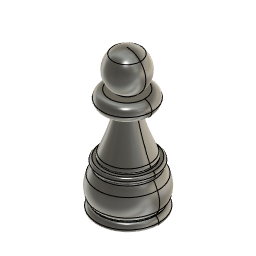
Pawn (Autodesk Fusion 360 design; units mm, degrees)
Autodesk Fusion 360 part; units mm, degrees
sketch "Chess Pieces_SVG" plane through (0, 0, 0) normal (0, 0, 1) x (1, 0, 0)
  spline S0 degree 3 poles (46.9799, 11.3155) (48.9199, 11.5598) (50.8372, 11.3177) (52.7479, 11.3837) knots 0 0 0 0 1 1 1 1
  spline S1 degree 3 poles (52.7479, 11.3837) (53.3742, 11.405) (53.207, 10.9554) (53.1909, 10.673) knots 0 0 0 0 1 1 1 1
  spline S2 degree 3 poles (53.1909, 10.673) (53.1249, 9.5941) (52.9877, 8.5188) (52.9166, 7.4399) knots 0 0 0 0 1 1 1 1
  spline S3 degree 3 poles (52.9166, 7.4399) (52.8748, 6.7959) (52.8682, 6.292) (53.8855, 6.4241) knots 0 0 0 0 1 1 1 1
  spline S4 degree 3 poles (53.8855, 6.4241) (54.6123, 6.5179) (55.4272, 6.4871) (56.1761, 6.4043) knots 0 0 0 0 1 1 1 1
  spline S5 degree 3 poles (56.1761, 6.4043) (57.3592, 6.273) (57.4626, 6.8172) (57.3159, 7.7443) knots 0 0 0 0 1 1 1 1
  spline S6 degree 3 poles (57.3159, 7.7443) (57.1728, 8.6465) (57.1384, 9.567) (56.9858, 10.4669) knots 0 0 0 0 1 1 1 1
  spline S7 degree 3 poles (56.9858, 10.4669) (56.8685, 11.1578) (57.153, 11.4043) (57.7802, 11.4035) knots 0 0 0 0 1 1 1 1
  spline S8 degree 3 poles (57.7802, 11.4035) (59.5097, 11.4013) (61.2406, 11.3984) (62.9687, 11.3881) knots 0 0 0 0 1 1 1 1
  spline S9 degree 3 poles (62.9687, 11.3881) (63.5547, 11.3852) (63.8899, 11.2568) (63.7586, 10.494) knots 0 0 0 0 1 1 1 1
  spline S10 degree 3 poles (63.7586, 10.494) (63.2848, 7.7443) (62.6225, 5.0099) (60.8673, 2.833) knots 0 0 0 0 1 1 1 1
  spline S11 degree 3 poles (60.8673, 2.833) (60.0011, 1.76) (59.1092, 0.4933) (57.0878, 0.5989) knots 0 0 0 0 1 1 1 1
  spline S12 degree 3 poles (57.0878, 0.5989) (52.31, 0.8483) (47.5109, 0.6612) (42.7207, 0.6392) knots 0 0 0 0 1 1 1 1
  spline S13 degree 3 poles (42.7207, 0.6392) (41.996, 0.6363) (41.3528, 0.7749) (40.8247, 1.3177) knots 0 0 0 0 1 1 1 1
  spline S14 degree 3 poles (40.8247, 1.3177) (38.3031, 3.9178) (37.1009, 7.1018) (36.7041, 10.6385) knots 0 0 0 0 1 1 1 1
  spline S15 degree 3 poles (36.7041, 10.6385) (36.6652, 10.9781) (36.5017, 11.4446) (37.1823, 11.4329) knots 0 0 0 0 1 1 1 1
  spline S16 degree 3 poles (37.1823, 11.4329) (38.9551, 11.4021) (40.7293, 11.4072) (42.5029, 11.4028) knots 0 0 0 0 1 1 1 1
  spline S17 degree 3 poles (42.5029, 11.4028) (43.1725, 11.4006) (43.4813, 11.1608) (43.3683, 10.4126) knots 0 0 0 0 1 1 1 1
  spline S18 degree 3 poles (43.3683, 10.4126) (43.2077, 9.3462) (43.1527, 8.2636) (43.0412, 7.1898) knots 0 0 0 0 1 1 1 1
  spline S19 degree 3 poles (43.0412, 7.1898) (42.995, 6.7593) (43.0295, 6.3346) (43.5752, 6.3881) knots 0 0 0 0 1 1 1 1
  spline S20 degree 3 poles (43.5752, 6.3881) (44.7245, 6.5025) (45.8834, 6.2033) (47.0327, 6.5077) knots 0 0 0 0 1 1 1 1
  spline S21 degree 3 poles (47.0327, 6.5077) (47.3239, 6.5854) (47.5476, 6.5473) (47.5058, 6.9477) knots 0 0 0 0 1 1 1 1
  spline S22 degree 3 poles (47.5058, 6.9477) (47.3532, 8.3883) (47.4259, 9.8545) (46.9799, 11.3155) knots 0 0 0 0 1 1 1 1
  spline S23 degree 3 poles (-16.835, 18.1287) (-19.0728, 18.0267) (-21.2409, 20.0423) (-21.3773, 22.3512) knots 0 0 0 0 1 1 1 1
  spline S24 degree 3 poles (-21.3773, 22.3512) (-21.5335, 24.9924) (-19.5642, 27.3219) (-17.0946, 27.415) knots 0 0 0 0 1 1 1 1
  spline S25 degree 3 poles (-17.0946, 27.415) (-14.4762, 27.5133) (-12.0484, 25.742) (-12.0902, 22.4458) knots 0 0 0 0 1 1 1 1
  spline S26 degree 3 poles (-12.0902, 22.4458) (-12.1151, 20.5205) (-13.7082, 18.1778) (-16.835, 18.1287) knots 0 0 0 0 1 1 1 1
  spline S27 degree 3 poles (-58.4766, 30.9107) (-57.8429, 30.1926) (-57.1527, 29.6858) (-56.3202, 29.355) knots 0 0 0 0 1 1 1 1
  spline S28 degree 3 poles (-56.3202, 29.355) (-56.0011, 29.2281) (-55.7122, 29.1797) (-55.443, 29.3382) knots 0 0 0 0 1 1 1 1
  spline S29 degree 3 poles (-55.443, 29.3382) (-55.0704, 29.5597) (-55.1701, 29.9689) (-55.2449, 30.2836) knots 0 0 0 0 1 1 1 1
  spline S30 degree 3 poles (-55.2449, 30.2836) (-55.4078, 30.9679) (-55.7408, 31.5686) (-56.2923, 32.041) knots 0 0 0 0 1 1 1 1
  spline S31 degree 3 poles (-56.2923, 32.041) (-56.7639, 32.4451) (-56.626, 32.7487) (-56.0928, 32.9739) knots 0 0 0 0 1 1 1 1
  spline S32 degree 3 poles (-56.0928, 32.9739) (-55.2889, 33.3128) (-54.4271, 33.4037) (-53.6027, 33.2886) knots 0 0 0 0 1 1 1 1
  spline S33 degree 3 poles (-53.6027, 33.2886) (-52.0837, 33.0751) (-52.0214, 32.8023) (-52.8986, 31.5701) knots 0 0 0 0 1 1 1 1
  spline S34 degree 3 poles (-52.8986, 31.5701) (-53.3313, 30.962) (-54.0589, 30.2198) (-53.3599, 29.5289) knots 0 0 0 0 1 1 1 1
  spline S35 degree 3 poles (-53.3599, 29.5289) (-52.6023, 28.7793) (-51.8387, 29.5912) (-51.2322, 30.0415) knots 0 0 0 0 1 1 1 1
  spline S36 degree 3 poles (-51.2322, 30.0415) (-50.1958, 30.8109) (-49.8841, 30.7889) (-49.6736, 29.5435) knots 0 0 0 0 1 1 1 1
  spline S37 degree 3 poles (-49.6736, 29.5435) (-49.5093, 28.5687) (-49.4088, 27.5617) (-49.876, 26.5899) knots 0 0 0 0 1 1 1 1
  spline S38 degree 3 poles (-49.876, 26.5899) (-50.1459, 26.0288) (-50.3219, 25.7904) (-50.806, 26.405) knots 0 0 0 0 1 1 1 1
  spline S39 degree 3 poles (-50.806, 26.405) (-51.2461, 26.9617) (-51.8607, 27.3219) (-52.5385, 27.5111) knots 0 0 0 0 1 1 1 1
  spline S40 degree 3 poles (-52.5385, 27.5111) (-53.3394, 27.7341) (-53.7281, 27.3373) (-53.5602, 26.5268) knots 0 0 0 0 1 1 1 1
  spline S41 degree 3 poles (-53.5602, 26.5268) (-53.3959, 25.7354) (-52.8597, 25.1611) (-52.3793, 24.5604) knots 0 0 0 0 1 1 1 1
  spline S42 degree 3 poles (-52.3793, 24.5604) (-52.0038, 24.091) (-52.0492, 23.8753) (-52.6837, 23.7118) knots 0 0 0 0 1 1 1 1
  spline S43 degree 3 poles (-52.6837, 23.7118) (-53.7531, 23.4353) (-54.8027, 23.2908) (-55.8706, 23.6604) knots 0 0 0 0 1 1 1 1
  spline S44 degree 3 poles (-55.8706, 23.6604) (-56.5732, 23.9039) (-56.9986, 24.1658) (-56.2278, 24.9102) knots 0 0 0 0 1 1 1 1
  spline S45 degree 3 poles (-56.2278, 24.9102) (-55.8009, 25.3224) (-55.5581, 25.9349) (-55.2713, 26.4777) knots 0 0 0 0 1 1 1 1
  spline S46 degree 3 poles (-55.2713, 26.4777) (-55.1173, 26.7696) (-55.1797, 27.1011) (-55.4004, 27.3453) knots 0 0 0 0 1 1 1 1
  spline S47 degree 3 poles (-55.4004, 27.3453) (-55.6307, 27.6006) (-55.9153, 27.6013) (-56.2432, 27.462) knots 0 0 0 0 1 1 1 1
  spline S48 degree 3 poles (-56.2432, 27.462) (-56.9121, 27.1774) (-57.6118, 26.9617) (-58.101, 26.3698) knots 0 0 0 0 1 1 1 1
  spline S49 degree 3 poles (-58.101, 26.3698) (-58.4898, 25.8997) (-58.7406, 26.0786) (-58.8954, 26.5679) knots 0 0 0 0 1 1 1 1
  spline S50 degree 3 poles (-58.8954, 26.5679) (-59.3538, 28.0194) (-59.4279, 29.4394) (-58.4766, 30.9107) knots 0 0 0 0 1 1 1 1
  spline S51 degree 3 poles (99.919, 0.4038) (97.4773, 2.1487) (95.6341, 4.3579) (94.363, 7.071) knots 0 0 0 0 1 1 1 1
  spline S52 degree 3 poles (94.363, 7.071) (94.0051, 7.8345) (93.6369, 8.6575) (92.9629, 9.1767) knots 0 0 0 0 1 1 1 1
  spline S53 degree 3 poles (92.9629, 9.1767) (92.25, 9.7254) (91.8524, 10.1882) (92.2155, 11.1725) knots 0 0 0 0 1 1 1 1
  spline S54 degree 3 poles (92.2155, 11.1725) (92.5111, 11.9727) (91.9778, 12.7692) (91.3492, 13.1631) knots 0 0 0 0 1 1 1 1
  spline S55 degree 3 poles (91.3492, 13.1631) (90.805, 13.5042) (90.3466, 12.8529) (89.9689, 12.4223) knots 0 0 0 0 1 1 1 1
  spline S56 degree 3 poles (89.9689, 12.4223) (89.5794, 11.98) (89.1525, 11.903) (88.5327, 12.0086) knots 0 0 0 0 1 1 1 1
  spline S57 degree 3 poles (88.5327, 12.0086) (85.3576, 12.5507) (82.3328, 12.0314) (79.4848, 10.5168) knots 0 0 0 0 1 1 1 1
  spline S58 degree 3 poles (79.4848, 10.5168) (76.8142, 9.0968) (75.0488, 6.8935) (73.8092, 4.1731) knots 0 0 0 0 1 1 1 1
  spline S59 degree 3 poles (73.8092, 4.1731) (72.2205, 0.6891) (71.4812, -2.9921) (71.234, -6.7687) knots 0 0 0 0 1 1 1 1
  spline S60 degree 3 poles (71.234, -6.7687) (70.9634, -10.9143) (71.1357, -15.0605) (71.9448, -19.1452) knots 0 0 0 0 1 1 1 1
  spline S61 degree 3 poles (71.9448, -19.1452) (72.379, -21.3368) (72.921, -23.5041) (73.9163, -25.5476) knots 0 0 0 0 1 1 1 1
  spline S62 degree 3 poles (73.9163, -25.5476) (74.2581, -26.2524) (74.6674, -26.606) (75.2769, -26.7262) knots 0 0 0 0 1 1 1 1
  line L0 (75.2769, -26.7262) -> (92.9848, -26.7262)
  spline S63 degree 3 poles (92.9848, -26.7262) (93.4601, -26.6272) (93.6552, -26.314) (93.7176, -25.7331) knots 0 0 0 0 1 1 1 1
  spline S64 degree 3 poles (93.7176, -25.7331) (93.9603, -23.5225) (94.2229, -21.3148) (94.5097, -19.1107) knots 0 0 0 0 1 1 1 1
  spline S65 degree 3 poles (94.5097, -19.1107) (94.5933, -18.4711) (94.4034, -18.0428) (93.9273, -17.5968) knots 0 0 0 0 1 1 1 1
  spline S66 degree 3 poles (93.9273, -17.5968) (91.7548, -15.5695) (89.7429, -13.4014) (88.32, -10.7522) knots 0 0 0 0 1 1 1 1
  spline S67 degree 3 poles (88.32, -10.7522) (86.889, -8.0846) (85.7712, -5.3238) (85.6707, -2.244) knots 0 0 0 0 1 1 1 1
  spline S68 degree 3 poles (85.6707, -2.244) (85.6546, -1.7716) (85.7595, -1.1423) (86.1636, -1.1064) knots 0 0 0 0 1 1 1 1
  spline S69 degree 3 poles (86.1636, -1.1064) (86.7049, -1.058) (86.5788, -1.7254) (86.6536, -2.1149) knots 0 0 0 0 1 1 1 1
  spline S70 degree 3 poles (86.6536, -2.1149) (87.1362, -4.6461) (88.5569, -5.4544) (91.102, -4.8412) knots 0 0 0 0 1 1 1 1
  spline S71 degree 3 poles (91.102, -4.8412) (93.3112, -4.3094) (95.5358, -3.9522) (97.3974, -5.9245) knots 0 0 0 0 1 1 1 1
  spline S72 degree 3 poles (97.3974, -5.9245) (97.6423, -6.1842) (98.4506, -6.8971) (99.1004, -5.8336) knots 0 0 0 0 1 1 1 1
  spline S73 degree 3 poles (99.1004, -5.8336) (99.6373, -4.9578) (100.3305, -4.1679) (100.7713, -3.2144) knots 0 0 0 0 1 1 1 1
  spline S74 degree 3 poles (100.7713, -3.2144) (101.5238, -1.5875) (101.3529, -0.6216) (99.919, 0.4038) knots 0 0 0 0 1 1 1 1
  line L1 (63.1256, -42.2624) -> (37.0606, -42.2624)
  spline S75 degree 3 poles (37.0606, -42.2624) (36.253, -42.5485) (35.832, -43.2511) (35.4088, -44.5662) knots 0 0 0 0 1 1 1 1
  spline S76 degree 3 poles (35.4088, -44.5662) (35.1081, -45.5014) (35.3692, -45.6166) (36.1687, -45.6144) knots 0 0 0 0 1 1 1 1
  spline S77 degree 3 poles (36.1687, -45.6144) (40.4983, -45.5982) (44.8279, -45.599) (49.1568, -45.6019) knots 0 0 0 0 1 1 1 1
  spline S78 degree 3 poles (49.1568, -45.6019) (54.1972, -45.6056) (59.2353, -45.6041) (64.2735, -45.6378) knots 0 0 0 0 1 1 1 1
  spline S79 degree 3 poles (64.2735, -45.6378) (65.0876, -45.6437) (65.169, -45.3056) (65.0179, -44.6381) knots 0 0 0 0 1 1 1 1
  spline S80 degree 3 poles (65.0179, -44.6381) (64.7048, -43.2585) (64.1495, -42.5323) (63.1256, -42.2624) knots 0 0 0 0 1 1 1 1
  spline S81 degree 3 poles (-9.7204, -27.3922) (-9.6412, -27.39) (-9.562, -27.3864) (-9.4828, -27.3819) knots 0 0 0 0 1 1 1 1
  spline S82 degree 3 poles (-9.4828, -27.3819) (-9.4828, -27.3856) (-9.4828, -27.3893) (-9.4828, -27.3922) knots 0 0 0 0 1 1 1 1
  line L2 (-9.4828, -27.3922) -> (-6.4902, -27.3922)
  spline S83 degree 3 poles (-6.4902, -27.3922) (-6.0927, -26.4563) (-6.9325, -25.981) (-7.2743, -25.3554) knots 0 0 0 0 1 1 1 1
  spline S84 degree 3 poles (-7.2743, -25.3554) (-9.9023, -20.5556) (-11.3949, -15.4251) (-12.0169, -9.9989) knots 0 0 0 0 1 1 1 1
  spline S85 degree 3 poles (-12.0169, -9.9989) (-12.1592, -8.7557) (-12.0425, -7.4707) (-12.4922, -6.1409) knots 0 0 0 0 1 1 1 1
  line L3 (-12.4922, -6.1409) -> (-21.2754, -6.1409)
  spline S86 degree 3 poles (-21.2754, -6.1409) (-21.4712, -6.3697) (-21.5394, -6.6815) (-21.56, -7.0724) knots 0 0 0 0 1 1 1 1
  spline S87 degree 3 poles (-21.56, -7.0724) (-21.7338, -10.3744) (-22.2787, -13.6259) (-23.0415, -16.8392) knots 0 0 0 0 1 1 1 1
  spline S88 degree 3 poles (-23.0415, -16.8392) (-23.9342, -20.6055) (-26.0055, -23.8782) (-27.4981, -27.3922) knots 0 0 0 0 1 1 1 1
  line L4 (-27.4981, -27.3922) -> (-9.7204, -27.3922)
  spline S89 degree 3 poles (-5.968, -27.8162) (-6.0443, -27.811) (-6.155, -27.8132) (-6.2621, -27.8088) knots 0 0 0 0 1 1 1 1
  line L5 (-6.2621, -27.8088) -> (-27.8971, -27.8088)
  spline S90 degree 3 poles (-27.8971, -27.8088) (-27.9741, -27.8257) (-28.0562, -27.8316) (-28.1376, -27.8323) knots 0 0 0 0 1 1 1 1
  spline S91 degree 3 poles (-28.1376, -27.8323) (-29.0031, -27.8404) (-29.3339, -28.4902) (-29.2965, -29.1269) knots 0 0 0 0 1 1 1 1
  spline S92 degree 3 poles (-29.2965, -29.1269) (-29.2488, -29.9183) (-28.6371, -30.1772) (-27.7995, -30.1742) knots 0 0 0 0 1 1 1 1
  spline S93 degree 3 poles (-27.7995, -30.1742) (-20.5837, -30.15) (-13.3672, -30.1698) (-6.1514, -30.1882) knots 0 0 0 0 1 1 1 1
  spline S94 degree 3 poles (-6.1514, -30.1882) (-5.426, -30.1896) (-4.76, -30.0261) (-4.6661, -29.2383) knots 0 0 0 0 1 1 1 1
  spline S95 degree 3 poles (-4.6661, -29.2383) (-4.5642, -28.3765) (-5.0614, -27.8697) (-5.968, -27.8162) knots 0 0 0 0 1 1 1 1
  line L6 (41.1782, -2.9745) -> (58.8041, -2.9745)
  spline S96 degree 3 poles (58.8041, -2.9745) (58.8781, -2.9665) (58.9508, -2.9599) (59.0241, -2.9481) knots 0 0 0 0 1 1 1 1
  spline S97 degree 3 poles (59.0241, -2.9481) (59.9871, -2.7992) (60.7734, -1.9176) (60.6392, -1.1401) knots 0 0 0 0 1 1 1 1
  spline S98 degree 3 poles (60.6392, -1.1401) (60.4712, -0.1646) (59.8867, 0.2996) (58.8664, 0.2952) knots 0 0 0 0 1 1 1 1
  spline S99 degree 3 poles (58.8664, 0.2952) (53.1557, 0.2659) (47.4449, 0.2534) (41.7349, 0.2534) knots 0 0 0 0 1 1 1 1
  spline S100 degree 3 poles (41.7349, 0.2534) (40.9839, 0.2534) (40.3597, 0.0701) (40.0465, -0.6458) knots 0 0 0 0 1 1 1 1
  spline S101 degree 3 poles (40.0465, -0.6458) (39.616, -1.6301) (40.1822, -2.6393) (41.1782, -2.9745) knots 0 0 0 0 1 1 1 1
  spline S102 degree 3 poles (59.6659, -16.058) (59.2441, -12.3526) (58.9089, -8.642) (58.5584, -4.9314) knots 0 0 0 0 1 1 1 1
  spline S103 degree 3 poles (58.5584, -4.9314) (58.4579, -3.865) (58.4051, -3.507) (57.8894, -3.3911) knots 0 0 0 0 1 1 1 1
  line L7 (57.8894, -3.3911) -> (42.4677, -3.3911)
  spline S104 degree 3 poles (42.4677, -3.3911) (42.2373, -3.4711) (42.0672, -3.6647) (42.0312, -4.1385) knots 0 0 0 0 1 1 1 1
  spline S105 degree 3 poles (42.0312, -4.1385) (41.8523, -6.6015) (41.5948, -9.0593) (41.3565, -11.5172) knots 0 0 0 0 1 1 1 1
  spline S106 degree 3 poles (41.3565, -11.5172) (40.9729, -15.4676) (40.5775, -19.4165) (40.18, -23.4565) knots 0 0 0 0 1 1 1 1
  spline S107 degree 3 poles (40.18, -23.4565) (42.2982, -23.4565) (44.4539, -23.4535) (46.611, -23.4565) knots 0 0 0 0 1 1 1 1
  spline S108 degree 3 poles (46.611, -23.4565) (50.7448, -23.4609) (54.8778, -23.4425) (59.0102, -23.4924) knots 0 0 0 0 1 1 1 1
  spline S109 degree 3 poles (59.0102, -23.4924) (59.993, -23.5049) (60.268, -23.1792) (60.1947, -22.2242) knots 0 0 0 0 1 1 1 1
  spline S110 degree 3 poles (60.1947, -22.2242) (60.0385, -20.1661) (59.8984, -18.0934) (59.6659, -16.058) knots 0 0 0 0 1 1 1 1
  line L8 (-64.3963, -26.9763) -> (-44.2056, -26.9763)
  spline S111 degree 3 poles (-44.2056, -26.9763) (-44.1359, -26.2238) (-44.6031, -25.6231) (-44.9134, -25.0349) knots 0 0 0 0 1 1 1 1
  spline S112 degree 3 poles (-44.9134, -25.0349) (-47.8142, -19.5361) (-49.5335, -13.7102) (-49.9669, -7.5059) knots 0 0 0 0 1 1 1 1
  spline S113 degree 3 poles (-49.9669, -7.5059) (-50.0792, -5.8959) (-50.1114, -5.5856) (-51.1735, -5.4492) knots 0 0 0 0 1 1 1 1
  line L9 (-51.1735, -5.4492) -> (-58.6922, -5.4492)
  spline S114 degree 3 poles (-58.6922, -5.4492) (-58.9497, -5.5204) (-59.1543, -5.6891) (-59.1565, -6.0976) knots 0 0 0 0 1 1 1 1
  spline S115 degree 3 poles (-59.1565, -6.0976) (-59.1587, -6.7159) (-59.3619, -7.3247) (-59.3736, -7.9151) knots 0 0 0 0 1 1 1 1
  spline S116 degree 3 poles (-59.3736, -7.9151) (-59.4381, -11.1314) (-60.1151, -14.239) (-60.8882, -17.3342) knots 0 0 0 0 1 1 1 1
  spline S117 degree 3 poles (-60.8882, -17.3342) (-61.6239, -20.2784) (-63.0849, -22.9386) (-64.2071, -25.7309) knots 0 0 0 0 1 1 1 1
  spline S118 degree 3 poles (-64.2071, -25.7309) (-64.3941, -26.1959) (-64.7191, -26.6646) (-64.3963, -26.9763) knots 0 0 0 0 1 1 1 1
  line L10 (-65.374, -29.7708) -> (-43.1949, -29.7708)
  spline S119 degree 3 poles (-43.1949, -29.7708) (-42.7805, -29.5999) (-42.5098, -29.22) (-42.4313, -28.7433) knots 0 0 0 0 1 1 1 1
  spline S120 degree 3 poles (-42.4313, -28.7433) (-42.3272, -28.1037) (-42.9543, -27.6211) (-43.6592, -27.4274) knots 0 0 0 0 1 1 1 1
  spline S121 degree 3 poles (-43.6592, -27.4274) (-43.7472, -27.4025) (-43.8755, -27.4135) (-43.987, -27.3929) knots 0 0 0 0 1 1 1 1
  line L11 (-43.987, -27.3929) -> (-64.9017, -27.3929)
  spline S122 degree 3 poles (-64.9017, -27.3929) (-64.9208, -27.3952) (-64.9406, -27.3959) (-64.9604, -27.3973) knots 0 0 0 0 1 1 1 1
  spline S123 degree 3 poles (-64.9604, -27.3973) (-65.7951, -27.4487) (-66.2799, -27.935) (-66.2564, -28.7271) knots 0 0 0 0 1 1 1 1
  spline S124 degree 3 poles (-66.2564, -28.7271) (-66.2373, -29.3352) (-65.8985, -29.6608) (-65.374, -29.7708) knots 0 0 0 0 1 1 1 1
  line L12 (-66.5674, -42.3248) -> (-42.8223, -42.3248)
  spline S125 degree 3 poles (-42.8223, -42.3248) (-42.314, -42.2052) (-41.9465, -41.9074) (-41.6509, -41.3067) knots 0 0 0 0 1 1 1 1
  spline S126 degree 3 poles (-41.6509, -41.3067) (-40.1246, -38.2101) (-40.5889, -35.2337) (-42.1504, -32.3475) knots 0 0 0 0 1 1 1 1
  spline S127 degree 3 poles (-42.1504, -32.3475) (-42.5553, -31.5994) (-42.7607, -30.5762) (-43.5858, -30.1874) knots 0 0 0 0 1 1 1 1
  line L13 (-43.5858, -30.1874) -> (-59.2379, -30.1874)
  spline S128 degree 3 poles (-59.2379, -30.1874) (-60.0528, -30.2124) (-60.8669, -30.227) (-61.6752, -30.1874) knots 0 0 0 0 1 1 1 1
  line L14 (-61.6752, -30.1874) -> (-64.4932, -30.1874)
  spline S129 degree 3 poles (-64.4932, -30.1874) (-65.6454, -30.4683) (-66.4698, -31.2502) (-67.1857, -32.5983) knots 0 0 0 0 1 1 1 1
  spline S130 degree 3 poles (-67.1857, -32.5983) (-68.7898, -35.6195) (-68.9159, -38.5086) (-67.4057, -41.5378) knots 0 0 0 0 1 1 1 1
  spline S131 degree 3 poles (-67.4057, -41.5378) (-67.1908, -41.9712) (-66.9246, -42.2148) (-66.5674, -42.3248) knots 0 0 0 0 1 1 1 1
  line L15 (-42.512, -42.7392) -> (-66.5989, -42.7392)
  spline S132 degree 3 poles (-66.5989, -42.7392) (-67.6221, -42.9335) (-68.3072, -43.8474) (-68.1319, -45.0239) knots 0 0 0 0 1 1 1 1
  spline S133 degree 3 poles (-68.1319, -45.0239) (-67.9602, -46.1857) (-66.9378, -45.4545) (-66.307, -45.6063) knots 0 0 0 0 1 1 1 1
  spline S134 degree 3 poles (-66.307, -45.6063) (-66.1258, -45.6518) (-65.9241, -45.6158) (-65.7312, -45.6158) knots 0 0 0 0 1 1 1 1
  spline S135 degree 3 poles (-65.7312, -45.6158) (-58.0277, -45.618) (-50.3227, -45.6283) (-42.6184, -45.5931) knots 0 0 0 0 1 1 1 1
  spline S136 degree 3 poles (-42.6184, -45.5931) (-42.1387, -45.5909) (-41.4309, -45.9364) (-41.1515, -45.321) knots 0 0 0 0 1 1 1 1
  spline S137 degree 3 poles (-41.1515, -45.321) (-40.8654, -44.6924) (-41.2021, -44.0521) (-41.5343, -43.4638) knots 0 0 0 0 1 1 1 1
  spline S138 degree 3 poles (-41.5343, -43.4638) (-41.7837, -43.023) (-42.1196, -42.825) (-42.512, -42.7392) knots 0 0 0 0 1 1 1 1
  line L16 (6.5148, -28.0846) -> (26.022, -28.0846)
  spline S139 degree 3 poles (26.022, -28.0846) (26.7576, -27.8235) (27.0576, -27.214) (26.8706, -26.5348) knots 0 0 0 0 1 1 1 1
  spline S140 degree 3 poles (26.8706, -26.5348) (26.6799, -25.8431) (26.0865, -25.4661) (25.2636, -25.4735) knots 0 0 0 0 1 1 1 1
  spline S141 degree 3 poles (25.2636, -25.4735) (21.7877, -25.5013) (18.3111, -25.4852) (14.8345, -25.483) knots 0 0 0 0 1 1 1 1
  spline S142 degree 3 poles (14.8345, -25.483) (12.285, -25.4823) (9.7354, -25.4691) (7.1859, -25.4749) knots 0 0 0 0 1 1 1 1
  spline S143 degree 3 poles (7.1859, -25.4749) (6.2346, -25.4779) (5.7425, -26.0412) (5.741, -26.9345) knots 0 0 0 0 1 1 1 1
  spline S144 degree 3 poles (5.741, -26.9345) (5.7388, -27.5763) (6.0358, -27.935) (6.5148, -28.0846) knots 0 0 0 0 1 1 1 1
  line L17 (38.6661, -26.6969) -> (40.1506, -26.6969)
  spline S145 degree 3 poles (40.1506, -26.6969) (40.1675, -26.6969) (40.1837, -26.6969) (40.2005, -26.6969) knots 0 0 0 0 1 1 1 1
  line L18 (40.2005, -26.6969) -> (61.3807, -26.6969)
  spline S146 degree 3 poles (61.3807, -26.6969) (62.4384, -26.5781) (63.0156, -26.0867) (62.9833, -25.3275) knots 0 0 0 0 1 1 1 1
  spline S147 degree 3 poles (62.9833, -25.3275) (62.9437, -24.3931) (62.2066, -23.8819) (60.8878, -23.8775) knots 0 0 0 0 1 1 1 1
  spline S148 degree 3 poles (60.8878, -23.8775) (59.1591, -23.8701) (57.4288, -23.8687) (55.7, -23.8643) knots 0 0 0 0 1 1 1 1
  spline S149 degree 3 poles (55.7, -23.8643) (51.5134, -23.8569) (47.3276, -23.8452) (43.1402, -23.8437) knots 0 0 0 0 1 1 1 1
  spline S150 degree 3 poles (43.1402, -23.8437) (41.8765, -23.8415) (40.6142, -23.8643) (39.3504, -23.8789) knots 0 0 0 0 1 1 1 1
  spline S151 degree 3 poles (39.3504, -23.8789) (38.3324, -23.8914) (37.83, -24.5508) (37.8234, -25.4273) knots 0 0 0 0 1 1 1 1
  spline S152 degree 3 poles (37.8234, -25.4273) (37.8182, -26.0705) (38.1013, -26.5297) (38.6661, -26.6969) knots 0 0 0 0 1 1 1 1
  spline S153 degree 3 poles (64.8793, -32.5367) (64.173, -30.8028) (63.0933, -29.2941) (62.2125, -27.6673) knots 0 0 0 0 1 1 1 1
  spline S154 degree 3 poles (62.2125, -27.6673) (61.944, -27.1715) (61.4944, -27.137) (61.0176, -27.1377) knots 0 0 0 0 1 1 1 1
  spline S155 degree 3 poles (61.0176, -27.1377) (59.6673, -27.1377) (58.3163, -27.1384) (56.966, -27.1384) knots 0 0 0 0 1 1 1 1
  spline S156 degree 3 poles (56.966, -27.1384) (55.6795, -27.1392) (54.3937, -27.1384) (53.108, -27.1384) knots 0 0 0 0 1 1 1 1
  spline S157 degree 3 poles (53.108, -27.1384) (53.108, -27.1297) (53.108, -27.1223) (53.108, -27.1135) knots 0 0 0 0 1 1 1 1
  line L19 (53.108, -27.1135) -> (39.5052, -27.1135)
  spline S158 degree 3 poles (39.5052, -27.1135) (39.335, -27.1487) (39.1832, -27.2279) (39.0629, -27.404) knots 0 0 0 0 1 1 1 1
  spline S159 degree 3 poles (39.0629, -27.404) (37.8916, -29.1173) (36.6594, -30.8065) (35.6729, -32.6255) knots 0 0 0 0 1 1 1 1
  spline S160 degree 3 poles (35.6729, -32.6255) (34.4663, -34.8515) (34.9013, -37.2177) (35.7132, -39.4635) knots 0 0 0 0 1 1 1 1
  spline S161 degree 3 poles (35.7132, -39.4635) (36.2743, -41.0163) (36.63, -41.5752) (37.6041, -41.7417) knots 0 0 0 0 1 1 1 1
  line L20 (37.6041, -41.7417) -> (63.1872, -41.7417)
  spline S162 degree 3 poles (63.1872, -41.7417) (63.4351, -41.6471) (63.6603, -41.4688) (63.8408, -41.1446) knots 0 0 0 0 1 1 1 1
  spline S163 degree 3 poles (63.8408, -41.1446) (65.3576, -38.4198) (66.1372, -35.6239) (64.8793, -32.5367) knots 0 0 0 0 1 1 1 1
  spline S164 degree 3 poles (-4.7835, -42.4612) (-3.6312, -42.0248) (-3.409, -40.7698) (-3.1075, -39.6946) knots 0 0 0 0 1 1 1 1
  spline S165 degree 3 poles (-3.1075, -39.6946) (-2.2376, -36.5891) (-3.4258, -33.8804) (-4.9507, -31.2598) knots 0 0 0 0 1 1 1 1
  spline S166 degree 3 poles (-4.9507, -31.2598) (-5.3277, -30.6107) (-5.7641, -30.4222) (-6.5276, -30.4265) knots 0 0 0 0 1 1 1 1
  spline S167 degree 3 poles (-6.5276, -30.4265) (-13.563, -30.4662) (-20.5984, -30.4625) (-27.6337, -30.417) knots 0 0 0 0 1 1 1 1
  spline S168 degree 3 poles (-27.6337, -30.417) (-28.3305, -30.4126) (-28.7831, -30.6547) (-29.0662, -31.1615) knots 0 0 0 0 1 1 1 1
  spline S169 degree 3 poles (-29.0662, -31.1615) (-29.6508, -32.2103) (-30.4414, -33.122) (-30.894, -34.267) knots 0 0 0 0 1 1 1 1
  spline S170 degree 3 poles (-30.894, -34.267) (-32.0653, -37.2279) (-31.546, -39.9058) (-29.8752, -42.4612) knots 0 0 0 0 1 1 1 1
  line L21 (-29.8752, -42.4612) -> (-4.7835, -42.4612)
  line L22 (-4.493, -42.8785) -> (-29.9911, -42.8785)
  spline S171 degree 3 poles (-29.9911, -42.8785) (-30.1803, -43.0326) (-30.3784, -43.1939) (-30.5683, -43.3685) knots 0 0 0 0 1 1 1 1
  spline S172 degree 3 poles (-30.5683, -43.3685) (-31.1434, -43.8937) (-31.2974, -44.6513) (-31.0942, -45.2843) knots 0 0 0 0 1 1 1 1
  spline S173 degree 3 poles (-31.0942, -45.2843) (-30.8999, -45.8938) (-30.1473, -45.5821) (-29.65, -45.5872) knots 0 0 0 0 1 1 1 1
  spline S174 degree 3 poles (-29.65, -45.5872) (-26.3355, -45.6195) (-23.021, -45.6224) (-19.7058, -45.618) knots 0 0 0 0 1 1 1 1
  spline S175 degree 3 poles (-19.7058, -45.618) (-14.4857, -45.6107) (-9.2664, -45.5711) (-4.0471, -45.5997) knots 0 0 0 0 1 1 1 1
  spline S176 degree 3 poles (-4.0471, -45.5997) (-3.0914, -45.6056) (-3.1141, -45.2777) (-3.2329, -44.4995) knots 0 0 0 0 1 1 1 1
  spline S177 degree 3 poles (-3.2329, -44.4995) (-3.3759, -43.5563) (-3.8483, -43.1147) (-4.493, -42.8785) knots 0 0 0 0 1 1 1 1
  line L23 (74.0652, -29.5464) -> (94.1723, -29.5464)
  spline S178 degree 3 poles (94.1723, -29.5464) (94.6586, -29.2405) (95.0518, -28.8305) (94.7936, -28.0861) knots 0 0 0 0 1 1 1 1
  spline S179 degree 3 poles (94.7936, -28.0861) (94.4753, -27.17) (93.6853, -27.1216) (92.888, -27.123) knots 0 0 0 0 1 1 1 1
  spline S180 degree 3 poles (92.888, -27.123) (92.7325, -27.123) (92.5793, -27.1289) (92.4238, -27.1274) knots 0 0 0 0 1 1 1 1
  spline S181 degree 3 poles (92.4238, -27.1274) (88.5716, -27.123) (84.718, -27.1113) (80.8651, -27.1135) knots 0 0 0 0 1 1 1 1
  spline S182 degree 3 poles (80.8651, -27.1135) (78.8576, -27.1142) (76.8502, -27.1436) (74.8427, -27.1487) knots 0 0 0 0 1 1 1 1
  spline S183 degree 3 poles (74.8427, -27.1487) (73.9354, -27.1494) (73.2753, -27.5536) (73.2701, -28.4711) knots 0 0 0 0 1 1 1 1
  spline S184 degree 3 poles (73.2701, -28.4711) (73.2672, -29.0873) (73.6009, -29.4012) (74.0652, -29.5464) knots 0 0 0 0 1 1 1 1
  spline S185 degree 3 poles (94.2758, -42.6996) (93.0516, -42.7003) (91.8275, -42.6996) (90.6033, -42.6996) knots 0 0 0 0 1 1 1 1
  spline S186 degree 3 poles (90.6033, -42.6996) (90.6033, -42.6966) (90.6033, -42.6952) (90.6033, -42.6922) knots 0 0 0 0 1 1 1 1
  line L24 (90.6033, -42.6922) -> (76.6477, -42.6922)
  spline S187 degree 3 poles (76.6477, -42.6922) (76.1483, -42.7275) (75.6495, -42.7568) (75.1559, -42.6922) knots 0 0 0 0 1 1 1 1
  line L25 (75.1559, -42.6922) -> (73.5437, -42.6922)
  spline S188 degree 3 poles (73.5437, -42.6922) (73.4814, -42.704) (73.4117, -42.704) (73.3362, -42.6922) knots 0 0 0 0 1 1 1 1
  line L26 (73.3347, -42.6922) -> (72.8704, -42.6922)
  spline S189 degree 3 poles (72.8704, -42.6922) (72.2536, -42.7964) (71.9316, -43.3318) (71.6741, -43.865) knots 0 0 0 0 1 1 1 1
  spline S190 degree 3 poles (71.6741, -43.865) (71.0881, -45.0723) (71.4849, -45.6232) (72.8125, -45.5953) knots 0 0 0 0 1 1 1 1
  spline S191 degree 3 poles (72.8125, -45.5953) (73.4286, -45.5813) (74.0454, -45.596) (74.6623, -45.596) knots 0 0 0 0 1 1 1 1
  spline S192 degree 3 poles (74.6623, -45.596) (81.5282, -45.5997) (88.3956, -45.6026) (95.2623, -45.5997) knots 0 0 0 0 1 1 1 1
  spline S193 degree 3 poles (95.2623, -45.5997) (95.6246, -45.599) (96.0456, -45.7127) (96.1791, -45.1552) knots 0 0 0 0 1 1 1 1
  spline S194 degree 3 poles (96.1791, -45.1552) (96.4527, -44.0191) (95.4427, -42.6974) (94.2758, -42.6996) knots 0 0 0 0 1 1 1 1
  line L27 (93.9941, -29.963) -> (74.286, -29.963)
  spline S195 degree 3 poles (74.286, -29.963) (73.8004, -30.1904) (73.4425, -30.6664) (73.0912, -31.2312) knots 0 0 0 0 1 1 1 1
  spline S196 degree 3 poles (73.0912, -31.2312) (72.7098, -31.8443) (72.4157, -32.4854) (72.0929, -33.1184) knots 0 0 0 0 1 1 1 1
  spline S197 degree 3 poles (72.0929, -33.1184) (70.714, -35.805) (70.8593, -38.488) (72.0665, -41.1975) knots 0 0 0 0 1 1 1 1
  spline S198 degree 3 poles (72.0665, -41.1975) (72.3057, -41.7365) (72.5902, -42.126) (73.0112, -42.2756) knots 0 0 0 0 1 1 1 1
  line L28 (73.0112, -42.2756) -> (73.9053, -42.2756)
  spline S199 degree 3 poles (73.9053, -42.2756) (73.909, -42.2756) (73.9127, -42.2742) (73.9141, -42.2734) knots 0 0 0 0 1 1 1 1
  spline S200 degree 3 poles (73.9141, -42.2734) (73.9149, -42.2727) (73.9149, -42.2705) (73.9149, -42.269) knots 0 0 0 0 1 1 1 1
  spline S201 degree 3 poles (73.9149, -42.269) (73.9185, -42.2705) (73.9207, -42.2727) (73.9229, -42.2734) knots 0 0 0 0 1 1 1 1
  spline S202 degree 3 poles (73.9229, -42.2734) (75.3781, -42.2734) (76.8333, -42.2734) (78.2885, -42.2734) knots 0 0 0 0 1 1 1 1
  spline S203 degree 2 poles (78.2885, -42.2734) (78.2885, -42.2742) (78.2885, -42.2756) knots 0 0 0 1 1 1
  line L29 (78.2885, -42.2756) -> (94.6872, -42.2756)
  spline S204 degree 3 poles (94.6872, -42.2756) (95.0246, -42.1744) (95.2696, -41.9478) (95.4508, -41.5833) knots 0 0 0 0 1 1 1 1
  spline S205 degree 3 poles (95.4508, -41.5833) (95.9869, -40.5109) (96.4322, -39.4247) (96.5253, -38.1866) knots 0 0 0 0 1 1 1 1
  spline S206 degree 3 poles (96.5253, -38.1866) (96.7541, -35.1134) (95.6114, -32.5081) (93.9941, -29.963) knots 0 0 0 0 1 1 1 1
  line L30 (73.9134, -42.2734) -> (73.9134, -42.2756)
  line L31 (73.9134, -42.2756) -> (73.9259, -42.2756)
  line L32 (73.9259, -42.2756) -> (73.9215, -42.2734)
  line L33 (73.9215, -42.2734) -> (73.9141, -42.2734)
  line L34 (73.9141, -42.2734) -> (73.9134, -42.2734)
  spline S207 degree 3 poles (21.9417, 0.0275) (21.3835, 0.5285) (21.6058, 0.7185) (21.9043, 1.1981) knots 0 0 0 0 1 1 1 1
  spline S208 degree 3 poles (21.9043, 1.1981) (23.4922, 3.7469) (24.0856, 6.3698) (22.5145, 9.212) knots 0 0 0 0 1 1 1 1
  spline S209 degree 3 poles (22.5145, 9.212) (21.1547, 11.672) (19.6247, 14.011) (17.9451, 16.2569) knots 0 0 0 0 1 1 1 1
  spline S210 degree 3 poles (17.9451, 16.2569) (17.6972, 16.5869) (17.5629, 16.8502) (17.6451, 17.1583) knots 0 0 0 0 1 1 1 1
  spline S211 degree 3 poles (17.6451, 17.1583) (18.2913, 17.5808) (18.7196, 18.3098) (18.7196, 19.1401) knots 0 0 0 0 1 1 1 1
  spline S212 degree 3 poles (18.7196, 19.1401) (18.7196, 20.4479) (17.6605, 21.5077) (16.352, 21.5077) knots 0 0 0 0 1 1 1 1
  spline S213 degree 3 poles (16.352, 21.5077) (15.0435, 21.5077) (13.9844, 20.4479) (13.9844, 19.1401) knots 0 0 0 0 1 1 1 1
  spline S214 degree 3 poles (13.9844, 19.1401) (13.9844, 18.315) (14.4076, 17.5888) (15.0472, 17.1656) knots 0 0 0 0 1 1 1 1
  spline S215 degree 3 poles (15.0472, 17.1656) (15.1059, 16.6287) (14.7303, 16.196) (14.3753, 15.7046) knots 0 0 0 0 1 1 1 1
  spline S216 degree 3 poles (14.3753, 15.7046) (14.1039, 15.329) (13.848, 14.9396) (13.548, 14.5875) knots 0 0 0 0 1 1 1 1
  spline S217 degree 3 poles (13.548, 14.5875) (12.9253, 13.8592) (12.8197, 13.1433) (13.3089, 12.261) knots 0 0 0 0 1 1 1 1
  spline S218 degree 3 poles (13.3089, 12.261) (13.848, 11.2847) (14.2543, 10.2322) (14.6988, 9.2046) knots 0 0 0 0 1 1 1 1
  spline S219 degree 3 poles (14.6988, 9.2046) (14.7963, 8.9794) (14.9892, 8.6567) (14.6196, 8.5086) knots 0 0 0 0 1 1 1 1
  spline S220 degree 3 poles (14.6196, 8.5086) (14.3108, 8.3853) (14.1259, 8.6479) (13.9947, 8.8914) knots 0 0 0 0 1 1 1 1
  spline S221 degree 3 poles (13.9947, 8.8914) (13.8868, 9.0953) (13.8318, 9.3308) (13.7115, 9.5273) knots 0 0 0 0 1 1 1 1
  spline S222 degree 3 poles (13.7115, 9.5273) (13.1592, 10.4244) (12.9935, 11.537) (12.2204, 12.3614) knots 0 0 0 0 1 1 1 1
  spline S223 degree 3 poles (12.2204, 12.3614) (11.8119, 11.8333) (11.3953, 11.4175) (11.1268, 10.9217) knots 0 0 0 0 1 1 1 1
  spline S224 degree 3 poles (11.1268, 10.9217) (10.2679, 9.3322) (9.0467, 7.924) (9.2, 5.8798) knots 0 0 0 0 1 1 1 1
  spline S225 degree 3 poles (9.2, 5.8798) (9.3394, 4.0418) (9.965, 2.4582) (10.964, 0.9744) knots 0 0 0 0 1 1 1 1
  spline S226 degree 3 poles (10.964, 0.9744) (11.1224, 0.7397) (11.2977, 0.6011) (11.0857, 0.285) knots 0 0 0 0 1 1 1 1
  spline S227 degree 3 poles (11.0857, 0.285) (10.1594, -1.0954) (10.1799, -1.7291) (11.5309, -2.1604) knots 0 0 0 0 1 1 1 1
  line L35 (11.5309, -2.1604) -> (21.4268, -2.1604)
  spline S228 degree 3 poles (21.4268, -2.1604) (21.4415, -2.1552) (21.4547, -2.1508) (21.4679, -2.1442) knots 0 0 0 0 1 1 1 1
  spline S229 degree 3 poles (21.4679, -2.1442) (22.4801, -1.6374) (22.7456, -0.6935) (21.9417, 0.0275) knots 0 0 0 0 1 1 1 1
  line L36 (5.8694, -42.0453) -> (26.2207, -42.0453)
  spline S230 degree 3 poles (26.2207, -42.0453) (26.732, -41.9368) (27.0737, -41.6383) (27.3591, -41.0596) knots 0 0 0 0 1 1 1 1
  spline S231 degree 3 poles (27.3591, -41.0596) (28.9631, -37.8037) (28.9917, -34.5948) (27.3862, -31.3206) knots 0 0 0 0 1 1 1 1
  spline S232 degree 3 poles (27.3862, -31.3206) (26.927, -30.3833) (26.2442, -29.5376) (25.9912, -28.5012) knots 0 0 0 0 1 1 1 1
  line L37 (25.9912, -28.5012) -> (8.8641, -28.5012)
  spline S233 degree 3 poles (8.8641, -28.5012) (8.7885, -28.5093) (8.7159, -28.5093) (8.6433, -28.5012) knots 0 0 0 0 1 1 1 1
  line L38 (8.6433, -28.5012) -> (7.2651, -28.5012)
  spline S234 degree 3 poles (7.2651, -28.5012) (6.3645, -28.7645) (5.8576, -29.6095) (5.2936, -30.5975) knots 0 0 0 0 1 1 1 1
  spline S235 degree 3 poles (5.2936, -30.5975) (3.3631, -33.9795) (3.1805, -37.3438) (4.7303, -40.874) knots 0 0 0 0 1 1 1 1
  spline S236 degree 3 poles (4.7303, -40.874) (5.0002, -41.4894) (5.3229, -41.9045) (5.8694, -42.0453) knots 0 0 0 0 1 1 1 1
  line L39 (26.473, -42.4612) -> (11.8595, -42.4612)
  spline S237 degree 3 poles (11.8595, -42.4612) (11.4583, -42.4957) (11.0454, -42.5191) (10.6317, -42.4612) knots 0 0 0 0 1 1 1 1
  line L40 (10.6317, -42.4612) -> (6.0447, -42.4612)
  spline S238 degree 3 poles (6.0447, -42.4612) (4.8476, -42.6292) (4.3746, -43.1617) (4.2264, -44.5105) knots 0 0 0 0 1 1 1 1
  spline S239 degree 3 poles (4.2264, -44.5105) (4.1435, -45.2762) (4.324, -45.6056) (5.2151, -45.5982) knots 0 0 0 0 1 1 1 1
  spline S240 degree 3 poles (5.2151, -45.5982) (9.756, -45.5586) (14.299, -45.6004) (18.8414, -45.6034) knots 0 0 0 0 1 1 1 1
  spline S241 degree 3 poles (18.8414, -45.6034) (21.5779, -45.6063) (24.3167, -45.5938) (27.0525, -45.5821) knots 0 0 0 0 1 1 1 1
  spline S242 degree 3 poles (27.0525, -45.5821) (27.4156, -45.5813) (27.8168, -45.7068) (27.9334, -45.1134) knots 0 0 0 0 1 1 1 1
  spline S243 degree 3 poles (27.9334, -45.1134) (28.1483, -44.0191) (27.4713, -42.8023) (26.473, -42.4612) knots 0 0 0 0 1 1 1 1
  spline S244 degree 3 poles (-8.5813, 17.203) (-10.0138, 16.4248) (-11.425, 16.3243) (-12.7503, 17.181) knots 0 0 0 0 1 1 1 1
  spline S245 degree 3 poles (-12.7503, 17.181) (-13.5381, 17.69) (-14.0155, 17.6453) (-14.8003, 17.1928) knots 0 0 0 0 1 1 1 1
  spline S246 degree 3 poles (-14.8003, 17.1928) (-16.1778, 16.3977) (-17.6484, 16.0412) (-19.0955, 17.25) knots 0 0 0 0 1 1 1 1
  spline S247 degree 3 poles (-19.0955, 17.25) (-19.4351, 17.5338) (-19.9207, 17.9167) (-20.5478, 17.4949) knots 0 0 0 0 1 1 1 1
  spline S248 degree 3 poles (-20.5478, 17.4949) (-22.1445, 16.4226) (-23.7948, 16.3992) (-25.5118, 17.3152) knots 0 0 0 0 1 1 1 1
  spline S249 degree 3 poles (-25.5118, 17.3152) (-26.7235, 17.9614) (-27.8971, 17.5309) (-28.6775, 16.2994) knots 0 0 0 0 1 1 1 1
  spline S250 degree 3 poles (-28.6775, 16.2994) (-29.2679, 15.3694) (-29.0435, 14.0924) (-28.0408, 13.3039) knots 0 0 0 0 1 1 1 1
  spline S251 degree 3 poles (-28.0408, 13.3039) (-24.0567, 10.1699) (-22.6924, 5.7845) (-22.1966, 1.0192) knots 0 0 0 0 1 1 1 1
  spline S252 degree 3 poles (-22.1966, 1.0192) (-22.0587, -0.3084) (-22.0462, -0.8211) (-22.5655, -1.036) knots 0 0 0 0 1 1 1 1
  line L41 (-22.5655, -1.036) -> (-24.6647, -1.036)
  spline S253 degree 3 poles (-24.6647, -1.036) (-25.96, -1.036) (-27.0103, -2.0863) (-27.0103, -3.3809) knots 0 0 0 0 1 1 1 1
  spline S254 degree 3 poles (-27.0103, -3.3809) (-27.0103, -4.605) (-26.0722, -5.6091) (-24.8759, -5.7162) knots 0 0 0 0 1 1 1 1
  spline S255 degree 3 poles (-24.8759, -5.7162) (-24.862, -5.7184) (-24.848, -5.7228) (-24.8341, -5.7265) knots 0 0 0 0 1 1 1 1
  line L42 (-24.8341, -5.7265) -> (-24.6647, -5.7265)
  line L43 (-24.6647, -5.7265) -> (-9.7615, -5.7265)
  line L44 (-9.7615, -5.7265) -> (-9.6984, -5.7265)
  spline S256 degree 3 poles (-9.6984, -5.7265) (-9.6867, -5.725) (-9.6764, -5.7228) (-9.6654, -5.7214) knots 0 0 0 0 1 1 1 1
  spline S257 degree 3 poles (-9.6654, -5.7214) (-9.2297, -5.7038) (-8.8248, -5.5688) (-8.4816, -5.3444) knots 0 0 0 0 1 1 1 1
  spline S258 degree 3 poles (-8.4816, -5.3444) (-8.0708, -5.1067) (-7.776, -4.7759) (-7.6403, -4.3755) knots 0 0 0 0 1 1 1 1
  spline S259 degree 3 poles (-7.6403, -4.3755) (-7.498, -4.0733) (-7.4166, -3.7366) (-7.4166, -3.3809) knots 0 0 0 0 1 1 1 1
  spline S260 degree 3 poles (-7.4166, -3.3809) (-7.4166, -2.0856) (-8.4662, -1.036) (-9.7615, -1.036) knots 0 0 0 0 1 1 1 1
  line L45 (-9.7615, -1.036) -> (-11.5012, -1.036)
  spline S261 degree 3 poles (-11.5012, -1.036) (-11.7051, -0.846) (-11.6919, -0.4602) (-11.6626, 0.3239) knots 0 0 0 0 1 1 1 1
  spline S262 degree 3 poles (-11.6626, 0.3239) (-11.6597, 0.4009) (-11.6707, 0.4786) (-11.6663, 0.5549) knots 0 0 0 0 1 1 1 1
  spline S263 degree 3 poles (-11.6663, 0.5549) (-11.3501, 5.5006) (-9.8861, 9.9219) (-5.9453, 13.2431) knots 0 0 0 0 1 1 1 1
  spline S264 degree 3 poles (-5.9453, 13.2431) (-5.434, 13.6736) (-4.936, 14.1922) (-4.9133, 14.9726) knots 0 0 0 0 1 1 1 1
  spline S265 degree 3 poles (-4.9133, 14.9726) (-4.8553, 16.9999) (-6.7433, 18.202) (-8.5813, 17.203) knots 0 0 0 0 1 1 1 1
  line L46 (-93.5625, -31.0119) -> (-74.2658, -31.0119)
  spline S266 degree 3 poles (-74.2658, -31.0119) (-73.8089, -30.8204) (-73.4773, -30.4786) (-73.5969, -29.8919) knots 0 0 0 0 1 1 1 1
  spline S267 degree 3 poles (-73.5969, -29.8919) (-73.7172, -29.3007) (-74.0142, -29.0381) (-74.3942, -28.9178) knots 0 0 0 0 1 1 1 1
  line L47 (-74.3942, -28.9178) -> (-93.2999, -28.9178)
  spline S268 degree 3 poles (-93.2999, -28.9178) (-93.759, -29.1159) (-93.9952, -29.5435) (-94.0084, -30.1728) knots 0 0 0 0 1 1 1 1
  spline S269 degree 3 poles (-94.0084, -30.1728) (-94.0187, -30.6591) (-93.8375, -30.8967) (-93.5625, -31.0119) knots 0 0 0 0 1 1 1 1
  line L48 (-94.2424, -42.6174) -> (-73.6057, -42.6174)
  spline S270 degree 3 poles (-73.6057, -42.6174) (-73.0453, -42.2947) (-72.7681, -41.6383) (-72.4967, -40.9583) knots 0 0 0 0 1 1 1 1
  spline S271 degree 3 poles (-72.4967, -40.9583) (-71.6085, -38.7418) (-71.9004, -36.5664) (-72.7717, -34.4445) knots 0 0 0 0 1 1 1 1
  spline S272 degree 3 poles (-72.7717, -34.4445) (-73.2162, -33.3619) (-73.6717, -32.2565) (-74.5607, -31.4285) knots 0 0 0 0 1 1 1 1
  line L49 (-74.5607, -31.4285) -> (-93.3116, -31.4285)
  spline S273 degree 3 poles (-93.3116, -31.4285) (-93.3769, -31.4659) (-93.4378, -31.515) (-93.4921, -31.5869) knots 0 0 0 0 1 1 1 1
  spline S274 degree 3 poles (-93.4921, -31.5869) (-95.5399, -34.3124) (-96.8565, -37.2118) (-95.6037, -40.7024) knots 0 0 0 0 1 1 1 1
  spline S275 degree 3 poles (-95.6037, -40.7024) (-95.1666, -41.9206) (-94.9098, -42.4201) (-94.2424, -42.6174) knots 0 0 0 0 1 1 1 1
  line L50 (-73.5507, -43.0333) -> (-94.6341, -43.0333)
  spline S276 degree 3 poles (-94.6341, -43.0333) (-95.3969, -43.2812) (-95.8377, -44.0426) (-95.7475, -44.9975) knots 0 0 0 0 1 1 1 1
  spline S277 degree 3 poles (-95.7475, -44.9975) (-95.6462, -46.0713) (-94.7742, -45.5777) (-94.3018, -45.5835) knots 0 0 0 0 1 1 1 1
  spline S278 degree 3 poles (-94.3018, -45.5835) (-90.0609, -45.6327) (-85.8193, -45.607) (-81.5784, -45.6026) knots 0 0 0 0 1 1 1 1
  spline S279 degree 3 poles (-81.5784, -45.6026) (-78.7348, -45.6011) (-75.8897, -45.5784) (-73.0461, -45.6026) knots 0 0 0 0 1 1 1 1
  spline S280 degree 3 poles (-73.0461, -45.6026) (-72.3375, -45.6099) (-72.1872, -45.3679) (-72.3317, -44.7085) knots 0 0 0 0 1 1 1 1
  spline S281 degree 3 poles (-72.3317, -44.7085) (-72.5378, -43.7631) (-72.8246, -43.2907) (-73.5507, -43.0333) knots 0 0 0 0 1 1 1 1
  spline S282 degree 3 poles (-80.2149, -13.6853) (-80.3888, -12.9423) (-80.4174, -12.6085) (-80.1518, -12.4604) knots 0 0 0 0 1 1 1 1
  line L51 (-80.1518, -12.4604) -> (-77.4351, -12.4604)
  spline S283 degree 3 poles (-77.4351, -12.4604) (-75.889, -12.4604) (-74.6355, -11.2069) (-74.6355, -9.66) knots 0 0 0 0 1 1 1 1
  spline S284 degree 3 poles (-74.6355, -9.66) (-74.6355, -8.1139) (-75.889, -6.8597) (-77.4351, -6.8597) knots 0 0 0 0 1 1 1 1
  line L52 (-77.4351, -6.8597) -> (-80.2545, -6.8597)
  spline S285 degree 3 poles (-80.2545, -6.8597) (-80.2809, -6.8509) (-80.3066, -6.8435) (-80.3323, -6.834) knots 0 0 0 0 1 1 1 1
  spline S286 degree 3 poles (-80.3323, -6.834) (-75.7166, -3.5371) (-76.2095, 1.7563) (-78.883, 4.6065) knots 0 0 0 0 1 1 1 1
  spline S287 degree 3 poles (-78.883, 4.6065) (-81.464, 7.3578) (-86.3225, 7.6629) (-89.2747, 4.5603) knots 0 0 0 0 1 1 1 1
  spline S288 degree 3 poles (-89.2747, 4.5603) (-91.5858, 2.1318) (-92.6691, -2.9921) (-87.785, -6.8597) knots 0 0 0 0 1 1 1 1
  line L53 (-87.785, -6.8597) -> (-90.7658, -6.8597)
  spline S289 degree 3 poles (-90.7658, -6.8597) (-92.3119, -6.8597) (-93.5661, -8.1139) (-93.5661, -9.66) knots 0 0 0 0 1 1 1 1
  spline S290 degree 3 poles (-93.5661, -9.66) (-93.5661, -11.2069) (-92.3119, -12.4604) (-90.7658, -12.4604) knots 0 0 0 0 1 1 1 1
  line L54 (-90.7658, -12.4604) -> (-88.129, -12.4604)
  spline S291 degree 3 poles (-88.129, -12.4604) (-87.6016, -12.635) (-87.683, -13.0948) (-87.9933, -14.3168) knots 0 0 0 0 1 1 1 1
  spline S292 degree 3 poles (-87.9933, -14.3168) (-89.139, -18.8371) (-90.325, -23.3457) (-92.1036, -27.6673) knots 0 0 0 0 1 1 1 1
  spline S293 degree 3 poles (-92.1036, -27.6673) (-92.2774, -28.0883) (-92.2393, -28.2731) (-92.0515, -28.3729) knots 0 0 0 0 1 1 1 1
  line L55 (-92.0515, -28.3729) -> (-75.5171, -28.3729)
  spline S294 degree 3 poles (-75.5171, -28.3729) (-75.2376, -28.166) (-75.366, -27.8998) (-75.6946, -27.1348) knots 0 0 0 0 1 1 1 1
  spline S295 degree 3 poles (-75.6946, -27.1348) (-77.5701, -22.7751) (-79.1279, -18.3083) (-80.2149, -13.6853) knots 0 0 0 0 1 1 1 1
  spline S296 degree 3 poles (-43.6628, 14.5963) (-43.0849, 15.6363) (-43.0379, 16.7402) (-43.3709, 17.8441) knots 0 0 0 0 1 1 1 1
  spline S297 degree 3 poles (-43.3709, 17.8441) (-43.9584, 19.7892) (-45.5222, 20.7779) (-47.8516, 20.7134) knots 0 0 0 0 1 1 1 1
  spline S298 degree 3 poles (-47.8516, 20.7134) (-48.8242, 20.6855) (-49.6787, 20.7493) (-49.6127, 22.0549) knots 0 0 0 0 1 1 1 1
  spline S299 degree 3 poles (-49.6127, 22.0549) (-49.5797, 22.7135) (-50.0439, 22.9607) (-50.55, 22.9622) knots 0 0 0 0 1 1 1 1
  spline S300 degree 3 poles (-50.55, 22.9622) (-53.1172, 22.971) (-55.6843, 22.9204) (-58.2521, 22.905) knots 0 0 0 0 1 1 1 1
  spline S301 degree 3 poles (-58.2521, 22.905) (-58.8968, 22.9006) (-59.554, 22.7106) (-59.5768, 22.0541) knots 0 0 0 0 1 1 1 1
  spline S302 degree 3 poles (-59.5768, 22.0541) (-59.6156, 20.9275) (-60.0733, 20.6034) (-61.1163, 20.7941) knots 0 0 0 0 1 1 1 1
  spline S303 degree 3 poles (-61.1163, 20.7941) (-61.4442, 20.8549) (-61.8043, 20.7544) (-62.1468, 20.7185) knots 0 0 0 0 1 1 1 1
  spline S304 degree 3 poles (-62.1468, 20.7185) (-65.8809, 20.3305) (-66.9847, 16.8458) (-65.2567, 13.9443) knots 0 0 0 0 1 1 1 1
  spline S305 degree 3 poles (-65.2567, 13.9443) (-63.7597, 11.4314) (-62.0243, 9.0609) (-60.3916, 6.6287) knots 0 0 0 0 1 1 1 1
  spline S306 degree 3 poles (-60.3916, 6.6287) (-60.143, 6.2583) (-60.0718, 5.8652) (-60.1005, 5.4192) knots 0 0 0 0 1 1 1 1
  spline S307 degree 3 poles (-60.1005, 5.4192) (-60.2163, 3.6508) (-60.3234, 1.8832) (-60.3924, 0.1134) knots 0 0 0 0 1 1 1 1
  spline S308 degree 3 poles (-60.3924, 0.1134) (-60.4048, -0.1998) (-60.4459, -0.4397) (-60.5611, -0.6113) knots 0 0 0 0 1 1 1 1
  line L56 (-60.5611, -0.6113) -> (-61.5615, -0.6113)
  spline S309 degree 3 poles (-61.5615, -0.6113) (-62.7827, -0.6113) (-63.7729, -1.6007) (-63.7729, -2.8212) knots 0 0 0 0 1 1 1 1
  spline S310 degree 3 poles (-63.7729, -2.8212) (-63.7729, -3.9302) (-62.9566, -4.8449) (-61.893, -5.0048) knots 0 0 0 0 1 1 1 1
  spline S311 degree 3 poles (-61.893, -5.0048) (-61.86, -5.0128) (-61.83, -5.0246) (-61.7969, -5.0319) knots 0 0 0 0 1 1 1 1
  line L57 (-61.7969, -5.0319) -> (-61.5615, -5.0319)
  line L58 (-61.5615, -5.0319) -> (-47.8238, -5.0319)
  line L59 (-47.8238, -5.0319) -> (-47.5216, -5.0319)
  spline S312 degree 3 poles (-47.5216, -5.0319) (-47.0822, -4.9475) (-46.717, -4.7788) (-46.4346, -4.5397) knots 0 0 0 0 1 1 1 1
  spline S313 degree 3 poles (-46.4346, -4.5397) (-46.4258, -4.5339) (-46.4177, -4.5265) (-46.4089, -4.5199) knots 0 0 0 0 1 1 1 1
  spline S314 degree 3 poles (-46.4089, -4.5199) (-46.3796, -4.4935) (-46.3495, -4.4686) (-46.3224, -4.4407) knots 0 0 0 0 1 1 1 1
  spline S315 degree 3 poles (-46.3224, -4.4407) (-45.8867, -4.0373) (-45.6131, -3.4623) (-45.6131, -2.8212) knots 0 0 0 0 1 1 1 1
  spline S316 degree 3 poles (-45.6131, -2.8212) (-45.6131, -1.6008) (-46.6033, -0.6113) (-47.8238, -0.6113) knots 0 0 0 0 1 1 1 1
  line L60 (-47.8238, -0.6113) -> (-48.6306, -0.6113)
  spline S317 degree 3 poles (-48.6306, -0.6113) (-48.7164, -0.502) (-48.7633, -0.3517) (-48.7714, -0.1412) knots 0 0 0 0 1 1 1 1
  spline S318 degree 3 poles (-48.7714, -0.1412) (-48.8484, 1.9045) (-48.921, 3.9501) (-49.02, 5.9942) knots 0 0 0 0 1 1 1 1
  spline S319 degree 3 poles (-49.02, 5.9942) (-49.0391, 6.3859) (-48.8411, 6.6353) (-48.6526, 6.9301) knots 0 0 0 0 1 1 1 1
  spline S320 degree 3 poles (-48.6526, 6.9301) (-47.0162, 9.5024) (-45.1474, 11.925) (-43.6628, 14.5963) knots 0 0 0 0 1 1 1 1
  spline S321 degree 3 poles (24.6783, -23.5929) (23.2935, -20.7448) (22.1133, -17.8301) (21.2369, -14.7701) knots 0 0 0 0 1 1 1 1
  spline S322 degree 3 poles (21.2369, -14.7701) (20.854, -13.4344) (20.8518, -12.032) (20.3626, -10.6355) knots 0 0 0 0 1 1 1 1
  line L61 (20.3626, -10.6355) -> (18.9147, -10.6355)
  spline S323 degree 3 poles (18.9147, -10.6355) (18.3426, -10.6553) (17.7698, -10.6517) (17.1977, -10.6355) knots 0 0 0 0 1 1 1 1
  line L62 (17.1977, -10.6355) -> (14.668, -10.6355)
  spline S324 degree 3 poles (14.668, -10.6355) (14.2528, -10.6957) (13.8281, -10.659) (13.4071, -10.6355) knots 0 0 0 0 1 1 1 1
  line L63 (13.4071, -10.6355) -> (12.7852, -10.6355)
  spline S325 degree 3 poles (12.7852, -10.6355) (12.3524, -10.6876) (12.1287, -10.9113) (12.0979, -11.5216) knots 0 0 0 0 1 1 1 1
  spline S326 degree 3 poles (12.0979, -11.5216) (12.0348, -12.756) (11.7649, -13.9713) (11.4077, -15.1588) knots 0 0 0 0 1 1 1 1
  spline S327 degree 3 poles (11.4077, -15.1588) (10.477, -18.2606) (9.2909, -21.2641) (7.8416, -24.162) knots 0 0 0 0 1 1 1 1
  spline S328 degree 3 poles (7.8416, -24.162) (7.5864, -24.6733) (7.3685, -25.1889) (8.2062, -25.2153) knots 0 0 0 0 1 1 1 1
  spline S329 degree 3 poles (8.2062, -25.2153) (9.775, -25.2637) (11.3461, -25.2226) (12.9164, -25.2146) knots 0 0 0 0 1 1 1 1
  spline S330 degree 3 poles (12.9164, -25.2146) (16.4891, -25.194) (20.0618, -25.1368) (23.6331, -25.1647) knots 0 0 0 0 1 1 1 1
  spline S331 degree 3 poles (23.6331, -25.1647) (25.3413, -25.1779) (25.4227, -25.1236) (24.6783, -23.5929) knots 0 0 0 0 1 1 1 1
  line L64 (10.3464, -10.2182) -> (10.5899, -10.2182)
  line L65 (10.5899, -10.2182) -> (11.3813, -10.2182)
  line L66 (11.3813, -10.2182) -> (15.1227, -10.2182)
  line L67 (15.1227, -10.2182) -> (20.2027, -10.2182)
  line L68 (20.2027, -10.2182) -> (21.6388, -10.2182)
  line L69 (21.6388, -10.2182) -> (22.3407, -10.2182)
  line L70 (22.3407, -10.2182) -> (22.4654, -10.2182)
  spline S332 degree 3 poles (22.4654, -10.2182) (22.483, -10.216) (22.4984, -10.2116) (22.5153, -10.2094) knots 0 0 0 0 1 1 1 1
  spline S333 degree 3 poles (22.5153, -10.2094) (23.49, -10.1206) (24.2528, -9.3028) (24.2528, -8.3046) knots 0 0 0 0 1 1 1 1
  spline S334 degree 3 poles (24.2528, -8.3046) (24.2528, -7.2484) (23.3969, -6.3917) (22.3407, -6.3917) knots 0 0 0 0 1 1 1 1
  line L71 (22.3407, -6.3917) -> (21.1877, -6.3917)
  spline S335 degree 3 poles (21.1877, -6.3917) (21.1562, -6.3103) (21.1349, -6.2076) (21.1253, -6.0771) knots 0 0 0 0 1 1 1 1
  spline S336 degree 3 poles (21.1253, -6.0771) (21.0395, -4.9101) (21.3667, -3.7366) (21.0373, -2.5755) knots 0 0 0 0 1 1 1 1
  line L72 (21.0373, -2.5755) -> (11.8434, -2.5755)
  spline S337 degree 3 poles (11.8434, -2.5755) (11.5317, -2.7831) (11.55, -3.1102) (11.5522, -3.4278) knots 0 0 0 0 1 1 1 1
  spline S338 degree 3 poles (11.5522, -3.4278) (11.5559, -4.0439) (11.5639, -4.6608) (11.5639, -5.2769) knots 0 0 0 0 1 1 1 1
  spline S339 degree 3 poles (11.5639, -5.2769) (11.5632, -5.7103) (11.5654, -6.1093) (11.3652, -6.3925) knots 0 0 0 0 1 1 1 1
  line L73 (11.3652, -6.3925) -> (10.3479, -6.3925)
  spline S340 degree 3 poles (10.3479, -6.3925) (9.2902, -6.3925) (8.4343, -7.2484) (8.4343, -8.3053) knots 0 0 0 0 1 1 1 1
  spline S341 degree 3 poles (8.4343, -8.3053) (8.4343, -9.3622) (9.288, -10.2182) (10.3464, -10.2182) knots 0 0 0 0 1 1 1 1
  line L74 (-84.0308, 6.7796) -> (-84.0308, -45.6068)
  constraint coincident S287 L74.start
  constraint coincident S278 L74.end
  constraint perpendicular L50 L74
  constraint perpendicular L48 L74
revolve "Revolve1" add sketch "Chess Pieces_SVG" angle 360 about axis through (-84.0308, 6.7796, 0) along (0, -1, 0) contours S282 L51 S283 S284 L52 S285 S286 S287 L55 S294 S295 L74 makes body 1
revolve "Revolve2" add sketch "Chess Pieces_SVG" angle 360 about axis through (-84.0308, 6.7796, 0) along (0, -1, 0) separate body contours L46 S266 S267 L47 L74 makes body 2
revolve "Revolve3" add sketch "Chess Pieces_SVG" angle 360 about axis through (-84.0308, 6.7796, 0) along (0, -1, 0) separate body contours L48 S270 S271 S272 L49 L74 makes body 3
revolve "Revolve4" add sketch "Chess Pieces_SVG" angle 360 about axis through (-84.0308, 6.7796, 0) along (0, -1, 0) separate body contours L50 S278 S279 S280 S281 L74 makes body 4
extrude "Extrude1" add 1 faces at (-86.4716, -28.3729, 1.8485) along direction (0, -1, 0) blind 1 on bodies 1 bodies 1 2
extrude "Extrude2" add 1 faces at (-86.0946, -31.0119, -0.1248) along direction (0, -1, 0) blind 2 on bodies 1 bodies 1 3
extrude "Extrude3" add 1 faces at (-81.6298, -42.6174, -3.1286) along direction (0, -1, 0) blind 2 on bodies 1 bodies 1 4
move_body "Move1" bodies 1 to x (0.999893, -0.010345, 0.010346) y (-0.010345, 0.000107, 0.999946) z (-0.010346, -0.999946, 0) at (-0.4796, -46.3534, 46.3559)
named bodies: "Pawn"
